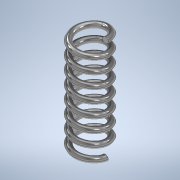
# Autodesk Inventor part: Peça14
Saved by Autodesk Inventor 2021 (Build 250183000, 183)
## iProperties
Created: 2020-11-15
Part Number: Peça14
Material: Liga de Nickel-Copper 400
Document SubType Name: Modeling
Designer: Bruno
Density: 8.83 g/cm^3
Appearance: Cromado - Preto polido
Author: Bruno
Autodesk Inventor part; units mm, degrees
ref_plane "YZ Plane" through (0, 0, 0) normal (1, 0, 0) x (0, 1, 0)
ref_plane "XZ Plane" through (0, 0, 0) normal (0, 1, 0) x (-1, 0, 0)
ref_plane "XY Plane" through (0, 0, 0) normal (0, 0, 1) x (1, 0, 0)
sketch "Esboço1" plane through (0, 0, 0) normal (0, 0, 1) x (1, 0, 0)
  circle A0 centre (0.21, 0) radius 0.04
  point P0 (0, 0)
  dimension "d3" = 0.08
  dimension "d4" = 0.21
  constraints: 1 centre point
  measures "d3" diameter of A0
  measures "d4" distance of A0.centre point (0, 0)
coil "Espiral1" sketch "Esboço1" operation add axis through (0, -10, 0) along (0, 1, 0) pitch 0.1744 turns 8 hand left
